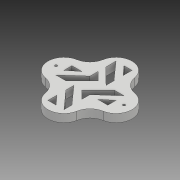
# Autodesk Inventor part: soporte_nuc_down
Saved by Autodesk Inventor 2018 (Build 220112000, 112)
## iProperties
Created: 2019-01-10
Part Number: soporte_nuc_down
Material: Genérico
Document SubType Name: Modeling
Designer: becar
Density: 1 g/cm^3
Appearance: Valor por defecto
Author: becar
Autodesk Inventor part; units mm, degrees
ref_plane "YZ Plane" through (0, 0, 0) normal (1, 0, 0) x (0, 1, 0)
ref_plane "XZ Plane" through (0, 0, 0) normal (0, 1, 0) x (-1, 0, 0)
ref_plane "XY Plane" through (0, 0, 0) normal (0, 0, 1) x (1, 0, 0)
sketch "Boceto1" plane through (0, 0, 0) normal (0, 0, 1) x (1, 0, 0)
  circle A0 centre (0, 0) radius 1.5
  line L0 (-10, 0) -> (-10, 20)
  line L1 (0, 0) -> (85, 0)
  circle A1 centre (85, 0) radius 1.5
  line L2 (42.5, 0) -> (42.5, 20)
  line L3 (42.5, 20) -> (-10, 20)
  line L4 (42.5, 20) -> (22.5, 20)
  line L5 (-10, 0) -> (-10, -20)
  line L6 (-10, -20) -> (22.5, -20)
  line L7 (22.5, -20) -> (22.5, -52.5)
  line L8 (22.5, -52.5) -> (42.5, -52.5)
  line L9 (42.5, -52.5) -> (62.5, -52.5)
  line L10 (62.5, -52.5) -> (62.5, -20)
  line L11 (62.5, -20) -> (85, -20)
  line L12 (85, -20) -> (95, -20)
  line L13 (95, -20) -> (95, 20)
  line L14 (95, 20) -> (62.5, 20)
  line L15 (62.5, 20) -> (62.5, 52.5)
  line L16 (62.5, 52.5) -> (22.5, 52.5)
  line L17 (22.5, 52.5) -> (22.5, 20)
  dimension "d0" = 3
  dimension "d1" = 10
  dimension "d2" = 20
  dimension "d3" = 85
  dimension "d4" = 3
  dimension "d5" = 20
  dimension "d6" = 20
  dimension "d7" = 32.5
  dimension "d8" = 20
  dimension "d9" = 20
  dimension "d10" = 10
  dimension "d11" = 32.5
  dimension "d12" = 40
  constraints: 36 end point, 8 perpendicular, 7 point on line, 2 centre point, 2 coincident, 2 horizontal, 2 vertical, 1 midpoint
  measures "d0" diameter of A0
  measures "d1" distance of L1.start L0.start
  measures "d2" distance of L0.start L0.end
  measures "d3" distance of L1.start L1.end
  measures "d4" diameter of A1
  measures "d5" distance of L2.end L4.end
  measures "d6" distance of L0.start L5.end
  measures "d7" distance of L6.end L7.end
  measures "d8" distance of L7.end L8.end
  measures "d9" distance of L8.end L9.end
  measures "d10" distance of L11.end L12.end
  measures "d11" distance of L14.end L15.end
  measures "d12" distance of L15.end L16.end
extrude "Extrusión1" add sketch "Boceto1" along normal blind 10
sketch "Boceto2" plane through (0, 0, 0) normal (0, 0, -1) x (-1, 0, 0)
  circle A0 centre (-85, 0) radius 1.5 projected
  circle A1 centre (-85, 0) radius 4
  circle A2 centre (0, 0) radius 4
  circle A3 centre (0, 0) radius 1.5 projected
  circle A4 centre (0, 0) radius 1.5
  dimension "d15" = 8
  dimension "d16" = 8
  constraints: 3 centre point, 3 coincident
  measures "d15" diameter of A1
  measures "d16" diameter of A2
extrude "Extrusión2" cut sketch "Boceto2" against normal blind 5
sketch "Boceto3" plane through (0, 0, 0) normal (0, 0, -1) x (-1, 0, 0)
  line L0 (-62.5, 52.5) -> (-22.5, 52.5) projected
  line L1 (-42.5, 52.5) -> (-52.5, 52.5)
  line L2 (-42.5, 52.5) -> (-32.5, 52.5)
  line L3 (-22.5, -52.5) -> (-62.5, -52.5) projected
  line L4 (-95, -20) -> (-95, 20) projected
  line L5 (-95, 20) -> (-95, 10)
  line L6 (9.9487, 10) -> (10, -9.9999)
  line L7 (10, 20) -> (10, -20) projected
  circle A0 centre (-85, 0) radius 4 projected
  line L8 (-81, 0) -> (-75, 0)
  line L9 (-75, 0) -> (-75, -10.3053)
  line L10 (-74.9213, 10) -> (-52.5, -10.1603)
  line L11 (-3.9534, -0.0578) -> (-9.9534, -0.0578)
  line L12 (-9.9534, -0.0578) -> (-9.9071, 9.942)
  line L13 (-9.9999, -10.109) -> (-32.5, 9.9984)
  line L14 (-22.407, 9.9999) -> (-9.9534, -0.0578)
  line L15 (-22.5, -10.0833) -> (-42.5257, 10)
  line L16 (-52.5, 52.5) -> (-52.5, 42.5)
  line L17 (-52.5, 20) -> (-32.5, 42.5)
  line L18 (-42.5, 42.5) -> (-52.5, 31.25)
  line L19 (-32.5, 29.8916) -> (-52.5, 10)
  line L20 (-52.5, -52.5) -> (-52.5, -42.5)
  line L21 (-52.5, -42.5) -> (-32.5, -42.5)
  line L22 (-42.5257, 10) -> (-32.4984, 19.9984)
  line L23 (-22.407, 9.9999) -> (-9.9534, -0.0578)
  line L24 (-9.9071, 9.942) -> (-22.407, 9.9999)
  line L25 (-75, -10.3053) -> (-63.7494, -10.3053)
  line L26 (-22.4744, -10.109) -> (-9.9999, -10.109)
  line L27 (-63.7494, -10.3053) -> (-62.5, -10.3053)
  line L28 (-62.5, -10.3053) -> (-75, 0)
  line L29 (-62.5, 10) -> (-42.5236, -10.1038)
  line L30 (-42.5236, -10.1038) -> (-32.5128, -0.0417)
  line L31 (-42.5257, 10) -> (-52.5118, -0.0519)
  line L32 (-62.5, 10) -> (-74.9213, 10)
  line L33 (-32.5, 9.9404) -> (-32.4984, 19.9984)
  line L34 (-42.5, -42.5) -> (-32.5, -31.25)
  line L35 (-52.5, -42.5) -> (-32.5, -20.0757)
  line L36 (-52.5, -20) -> (-42.5236, -10.1038)
  line L37 (-32.5, -10.1037) -> (-52.5, -32.528)
  line L38 (-42.5, -42.5) -> (-32.5, -42.5)
  line L39 (-32.5, -31.25) -> (-32.5, -42.5)
  line L40 (-32.5, -10.1037) -> (-32.5, -20.0757)
  line L41 (-52.5, -32.528) -> (-52.5, -42.5)
  line L42 (-52.5, 42.5) -> (-52.5, 31.25)
  line L43 (-52.5, 42.5) -> (-42.5, 42.5)
  line L44 (-32.5, 42.5) -> (-32.5, 29.8916)
  line L45 (-52.5, 10) -> (-52.5, 20)
  line L46 (-52.5, -20) -> (-52.5, -10.1603)
  line L47 (-42.5257, 10) -> (-22.4744, -10.109)
  line L48 (-22.4744, -10.109) -> (-9.9999, -10.109)
  line L49 (-9.9999, -10.109) -> (-32.5, 9.9984)
  line L50 (-32.5, 9.9984) -> (-32.4984, 19.9984)
  line L51 (-42.5257, 10) -> (-32.4984, 19.9984)
  point P0 (0, 0)
  dimension "d19" = 10
  dimension "d20" = 10
  dimension "d21" = 10
  dimension "d22" = 20
  dimension "d23" = 6
  dimension "d24" = 6
  dimension "d25" = 10
  dimension "d26" = 10
  constraints: 96 end point, 8 horizontal, 8 point on line, 4 midpoint, 3 collinear, 3 parallel, 3 vertical, 2 perpendicular, 1 horizontal alignment, 1 other
  measures "d19" distance of L1.start L1.end
  measures "d20" distance of L1.start L2.end
  measures "d21" distance of L4.end L5.end
  measures "d22" distance of L6.start L6.end
  measures "d23" distance of L8.start L8.end
  measures "d24" distance of L11.start L11.end
  measures "d25" distance of L1.end L16.end
  measures "d26" distance of L20.start L20.end
extrude "Extrusión3" cut sketch "Boceto3" against normal blind 10 contours L28 L27 L25 L9 | L32 L29 L36 L46 L10 | L22 L33 L13 L26 L47 L15 | L14 L24 L12 | L17 L44 L19 L45 | L18 L42 L43 | L34 L39 L21 | L41 L37 L40 L35
fillet "Empalme1" radius 20 8 edges at (95, -20, 5) (62.5, -52.5, 5) (22.5, -52.5, 5) (-10, -20, 5) (-10, 20, 5) (22.5, 52.5, 5) (95, 20, 5) (62.5, 52.5, 5)
fillet "Empalme2" radius 20 4 edges at (62.5, -20, 5) (62.5, 20, 5) (22.5, 20, 5) (22.5, -20, 5)
